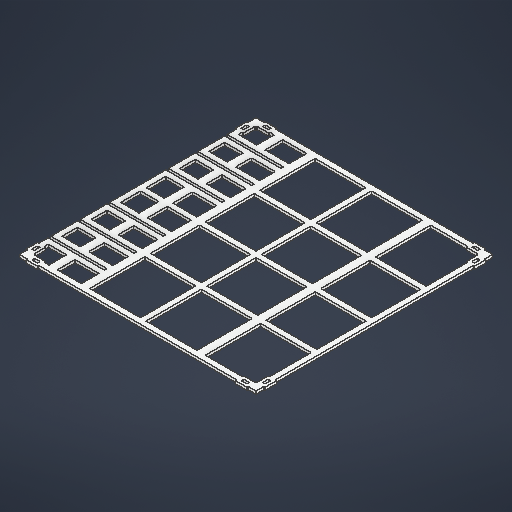
# Autodesk Inventor part: seat
Saved by Autodesk Inventor 2027.1 (Build 311270010, 270A)
## iProperties
Created: 2025-09-19
Part Number: seat
Material: Foam Core Board
Document SubType Name: Modeling
Designer: Nick
Density: 0.141998 g/cm^3
Appearance: Default(1)
Mass: 39.809 g
Surface Area: 1606.94 cm^2
Volume: 280.349 cm^3
Author: Nick
Autodesk Inventor part; units mm, degrees
ref_plane "YZ Plane" through (0, 0, 0) normal (1, 0, 0) x (0, 1, 0)
ref_plane "XZ Plane" through (0, 0, 0) normal (0, 1, 0) x (-1, 0, 0)
ref_plane "XY Plane" through (0, 0, 0) normal (0, 0, 1) x (1, 0, 0)
sketch "Sketch11" plane through (0, 0, 0) normal (0, 1, 0) x (-1, 0, 0)
  line L0 (0, 0) -> (420.5, 0)
  line L1 (420.5, 0) -> (420.5, -420.5)
  line L2 (420.5, -420.5) -> (0, -420.5)
  line L3 (0, -420.5) -> (0, 0)
  line L4 (420.5, 0) -> (410.5, 0)
  line L5 (410.5, 0) -> (410.5, -10)
  line L6 (410.5, -10) -> (420.5, -10)
  line L7 (420.5, -10) -> (420.5, 0)
  line L8 (0, -420.5) -> (10, -420.5)
  line L9 (10, -420.5) -> (10, -410.5)
  line L10 (10, -410.5) -> (0, -410.5)
  line L11 (0, -410.5) -> (0, -420.5)
  line L12 (10, -410.5) -> (410.5, -410.5)
  line L13 (410.5, -410.5) -> (410.5, -10)
  line L14 (410.5, -10) -> (10, -10)
  line L15 (10, -10) -> (10, -410.5)
  line L16 (0, -46.5229) -> (115, -46.5229)
  line L17 (115, -10) -> (100, -10)
  line L18 (100, -10) -> (100, -410.5)
  line L19 (100, -410.5) -> (115, -410.5)
  line L20 (115, -410.5) -> (115, -10)
  line L21 (210.25, 0) -> (210.25, -567.6903)
  line L22 (305.5, -10) -> (320.5, -10)
  line L23 (320.5, -10) -> (320.5, -410.5)
  line L24 (320.5, -410.5) -> (305.5, -410.5)
  line L25 (305.5, -410.5) -> (305.5, -10)
  line L26 (420.5, -210.25) -> (420.5, -205.25)
  line L27 (420.5, -205.25) -> (0, -205.25)
  line L28 (0, -205.25) -> (0, -215.25)
  line L29 (0, -215.25) -> (420.5, -215.25)
  line L30 (420.5, -215.25) -> (420.5, -205.25)
  line L31 (210.25, -420.5) -> (215.25, -420.5)
  line L32 (215.25, -420.5) -> (205.25, -420.5)
  line L33 (205.25, -420.5) -> (205.25, -10)
  line L34 (205.25, -10) -> (215.25, -10)
  line L35 (215.25, -10) -> (215.25, -420.5)
  point P0 (305.5, -46.5229)
  point P1 (410.5, -205.25)
  point P2 (320.5, -205.25)
  point P3 (10, -205.25)
  point P4 (205.25, -205.25)
  point P5 (410.5, -215.25)
  point P6 (320.5, -215.25)
  point P7 (305.5, -205.25)
  point P8 (215.25, -205.25)
  point P9 (305.5, -215.25)
  point P10 (215.25, -410.5)
  point P11 (215.25, -215.25)
  point P12 (10, -215.25)
  point P13 (205.25, -215.25)
  point P14 (205.25, -410.5)
  point P15 (100, -205.25)
  point P16 (115, -205.25)
  point P17 (115, -215.25)
  point P18 (100, -215.25)
  dimension "d88" = 420.5
  dimension "d89" = 420.5
  dimension "d90" = 10
  dimension "d91" = 10
  dimension "d92" = 10
  dimension "d93" = 10
  dimension "d94" = 115
  dimension "d95" = 15
  dimension "d96" = 5
  dimension "d97" = 10
  dimension "d98" = 5
  dimension "d99" = 10
  constraints: 72 end point, 14 parallel, 8 horizontal, 8 point on line, 7 perpendicular, 5 symmetric about line, 3 midpoint, 1 vertical
  measures "d88" distance of L1.end L2.end
  measures "d89" distance of L0.end L1.end
  measures "d90" distance of L6.end L5.end
  measures "d91" distance of L5.end L4.end
  measures "d92" distance of L10.end L9.end
  measures "d93" distance of L9.end L8.end
  measures "d94" distance of L16.start L16.end
  measures "d95" distance of L19.end L18.end
  measures "d96" distance of L26.start L26.end
  measures "d97" distance of L28.end L27.end
  measures "d98" distance of L31.start L31.end
  measures "d99" distance of L33.end L34.end
extrude "Extrusion12" add sketch "Sketch11" along normal blind 5 contours L0 L21 L14 L15 L16 L3 | L0 L5 L14 L21 | L16 L15 L27 L3 | L0 L1 L6 L5 | L21 L27 L33 L14 | L14 L35 L27 L21 | L27 L15 L29 L3 | L6 L1 L27 L13 | L27 L35 L29 L21 | L21 L29 L33 L27 | L29 L15 L10 L3 | L27 L18 L29 L15 | L18 L14 L20 L16 | L16 L20 L27 L18 | L27 L1 L29 L13 | L13 L29 L23 L27 | L23 L27 L25 L14 | L27 L25 L29 L35 | L33 L29 L20 L27 | L29 L35 L12 L21 | L21 L12 L33 L29 | L10 L9 L2 L3 | L27 L20 L29 L18 | L29 L1 L2 L35 L12 L13 | L23 L29 L25 L27 | L21 L2 L33 L12 | L12 L35 L2 L21 | L12 L33 L2 L9 | L29 L20 L12 L18 | L23 L12 L25 L29
sketch "Sketch12" plane through (0, 5, 0) normal (0, 1, 0) x (1, 0, 0)
  line L0 (-420.5, 420.5) -> (-420.5, 0) projected
  line L1 (-420.5, 0) -> (-420.5, 51.25)
  line L2 (-420.5, 51.25) -> (-320.5, 51.25)
  line L3 (-320.5, 51.25) -> (-320.5, 55.75)
  line L4 (-320.5, 55.75) -> (-420.5, 55.75)
  line L5 (-420.5, 51.25) -> (-420.5, 41.25)
  line L6 (-420.5, 41.25) -> (-320.5, 41.25)
  line L7 (-320.5, 41.25) -> (-320.5, 51.25)
  line L8 (-320.5, 205.25) -> (-320.5, 10) projected
  line L9 (-320.5, 55.75) -> (-320.5, 65.75)
  line L10 (-320.5, 65.75) -> (-420.5, 65.75)
  line L11 (-420.5, 65.75) -> (-420.5, 55.75)
  line L12 (-420.5, 55.75) -> (-420.5, 51.25)
  line L13 (-320.5, 51.25) -> (-320.5, 55.75)
  line L14 (-370.5, 10) -> (-378, 10)
  line L15 (-320.5, 10) -> (-410.5, 10) projected
  line L16 (-410.5, 410.5) -> (-320.5, 410.5) projected
  line L17 (-378, 10) -> (-363, 10)
  line L18 (-363, 10) -> (-363, 410.5)
  line L19 (-363, 410.5) -> (-378, 410.5)
  line L20 (-378, 410.5) -> (-378, 10)
  line L21 (-320.5, 103.5) -> (-320.5, 108)
  line L22 (-320.5, 103.5) -> (-320.5, 108)
  line L23 (-320.5, 93.5) -> (-320.5, 103.5)
  line L24 (-320.5, 108) -> (-320.5, 118)
  line L25 (-420.5, 103.5) -> (-320.5, 103.5)
  line L26 (-420.5, 108) -> (-420.5, 103.5)
  line L27 (-320.5, 108) -> (-420.5, 108)
  line L28 (-420.5, 103.5) -> (-420.5, 93.5)
  line L29 (-420.5, 93.5) -> (-320.5, 93.5)
  line L30 (-420.5, 118) -> (-420.5, 108)
  line L31 (-320.5, 118) -> (-420.5, 118)
  line L32 (-320.5, 155.75) -> (-320.5, 160.25)
  line L33 (-320.5, 155.75) -> (-320.5, 160.25)
  line L34 (-320.5, 145.75) -> (-320.5, 155.75)
  line L35 (-320.5, 160.25) -> (-320.5, 170.25)
  line L36 (-420.5, 155.75) -> (-320.5, 155.75)
  line L37 (-420.5, 160.25) -> (-420.5, 155.75)
  line L38 (-320.5, 160.25) -> (-420.5, 160.25)
  line L39 (-420.5, 155.75) -> (-420.5, 145.75)
  line L40 (-420.5, 145.75) -> (-320.5, 145.75)
  line L41 (-420.5, 170.25) -> (-420.5, 160.25)
  line L42 (-320.5, 170.25) -> (-420.5, 170.25)
  line L43 (-420.5, 210.25) -> (40.6434, 210.25)
  line L44 (-420.5, 420.5) -> (-420.5, 369.25)
  line L45 (-420.5, 369.25) -> (-320.5, 369.25)
  line L46 (-320.5, 369.25) -> (-320.5, 364.75)
  line L47 (-320.5, 364.75) -> (-420.5, 364.75)
  line L48 (-420.5, 369.25) -> (-420.5, 379.25)
  line L49 (-420.5, 379.25) -> (-320.5, 379.25)
  line L50 (-320.5, 379.25) -> (-320.5, 369.25)
  line L51 (-320.5, 364.75) -> (-320.5, 354.75)
  line L52 (-320.5, 354.75) -> (-420.5, 354.75)
  line L53 (-420.5, 354.75) -> (-420.5, 364.75)
  line L54 (-420.5, 364.75) -> (-420.5, 369.25)
  line L55 (-320.5, 369.25) -> (-320.5, 364.75)
  line L56 (-370.5, 410.5) -> (-378, 410.5)
  line L57 (-320.5, 410.5) -> (-410.5, 410.5)
  line L58 (-378, 410.5) -> (-363, 410.5)
  line L59 (-320.5, 317) -> (-320.5, 312.5)
  line L60 (-320.5, 317) -> (-320.5, 312.5)
  line L61 (-320.5, 327) -> (-320.5, 317)
  line L62 (-320.5, 312.5) -> (-320.5, 302.5)
  line L63 (-420.5, 317) -> (-320.5, 317)
  line L64 (-420.5, 312.5) -> (-420.5, 317)
  line L65 (-320.5, 312.5) -> (-420.5, 312.5)
  line L66 (-420.5, 317) -> (-420.5, 327)
  line L67 (-420.5, 327) -> (-320.5, 327)
  line L68 (-420.5, 302.5) -> (-420.5, 312.5)
  line L69 (-320.5, 302.5) -> (-420.5, 302.5)
  line L70 (-320.5, 264.75) -> (-320.5, 260.25)
  line L71 (-320.5, 264.75) -> (-320.5, 260.25)
  line L72 (-320.5, 274.75) -> (-320.5, 264.75)
  line L73 (-320.5, 260.25) -> (-320.5, 250.25)
  line L74 (-420.5, 264.75) -> (-320.5, 264.75)
  line L75 (-420.5, 260.25) -> (-420.5, 264.75)
  line L76 (-320.5, 260.25) -> (-420.5, 260.25)
  line L77 (-420.5, 264.75) -> (-420.5, 274.75)
  line L78 (-420.5, 274.75) -> (-320.5, 274.75)
  line L79 (-420.5, 250.25) -> (-420.5, 260.25)
  line L80 (-320.5, 250.25) -> (-420.5, 250.25)
  line L81 (-420.5, 274.75) -> (-420.5, 250.25)
  line L82 (-420.5, 274.75) -> (-378, 274.75)
  line L83 (-378, 264.75) -> (-420.5, 264.75)
  line L84 (-378, 260.25) -> (-420.5, 260.25)
  line L85 (-378, 312.5) -> (-420.5, 312.5)
  line L86 (-420.5, 317) -> (-378, 317)
  line L87 (-410.5, 215.25) -> (-410.5, 410.5) projected
  line L88 (-410.5, 302.5) -> (-410.5, 274.75)
  point P0 (0, 0)
  point P1 (-363, 93.5)
  point P2 (-363, 103.5)
  point P3 (-363, 108)
  point P4 (-363, 118)
  point P5 (-363, 145.75)
  point P6 (-363, 155.75)
  point P7 (-363, 160.25)
  point P8 (-363, 170.25)
  point P9 (-378, 170.25)
  point P10 (-378, 145.75)
  point P11 (-378, 118)
  point P12 (-378, 108)
  point P13 (-378, 103.5)
  point P14 (-378, 93.5)
  point P15 (-378, 55.75)
  point P16 (-378, 51.25)
  point P17 (-363, 51.25)
  point P18 (-363, 55.75)
  point P19 (-378, 354.75)
  point P20 (-378, 364.75)
  point P21 (-378, 379.25)
  point P22 (-378, 369.25)
  point P23 (-363, 379.25)
  point P24 (-363, 369.25)
  point P25 (-363, 364.75)
  point P26 (-363, 354.75)
  point P27 (-363, 312.5)
  point P28 (-363, 302.5)
  point P29 (-363, 327)
  point P30 (-363, 317)
  point P31 (-363, 260.25)
  point P32 (-363, 250.25)
  point P33 (-363, 274.75)
  point P34 (-363, 264.75)
  point P35 (-378, 250.25)
  point P36 (-378, 327)
  point P37 (-378, 302.5)
  dimension "d102" = 51.25
  dimension "d103" = 100
  dimension "d104" = 4.5
  dimension "d105" = 10
  dimension "d106" = 10
  dimension "d111" = 7.5
  dimension "d112" = 15
  dimension "d115" = 52.25
  constraints: 164 end point, 27 point on line, 25 symmetric about line, 21 collinear, 16 vertical alignment, 9 parallel, 5 perpendicular, 3 horizontal, 15 other
  measures "d102" distance of L1.start L1.end
  measures "d103" distance of L1.end L2.end
  measures "d104" distance of L2.end L3.end
  measures "d105" distance of L1.end L5.end
  measures "d106" distance of L3.end L9.end
  measures "d111" distance of L14.start L14.end
  measures "d112" distance of L19.end L19.start
  measures "d115" distance of L3.end L21.end
extrude "Extrusion13" add sketch "Sketch12" against normal blind 5 contours L10 L20 L4 L0 | L10 L18 L4 L20 | L2 L20 L6 L0 | L10 L8 L4 L18 | L2 L18 L6 L20 | L2 L7 L6 L18
extrude "Extrusion14" cut sketch "Sketch12" against normal blind 5 contours L38 L20 L36 L0 | L38 L18 L36 L20 | L38 L8 L36 L18 | L27 L20 L25 L0 | L27 L18 L25 L20 | L27 L8 L25 L18 | L4 L20 L2 L0 | L4 L18 L2 L20 | L4 L3 L2 L18
extrude "Extrusion15" add sketch "Sketch12" against normal blind 5 contours L49 L87 L45 L0 | L49 L20 L45 L87 | L47 L87 L52 L0 | L49 L18 L45 L20 | L20 L16 L18 L49 | L47 L20 L52 L87 | L45 L18 L47 L20 | L49 L50 L45 L18 | L67 L87 L63 L0 | L47 L18 L52 L20 | L63 L87 L65 L0 | L67 L20 L63 L87 | L52 L18 L67 L20 | L47 L51 L52 L18 | L65 L87 L69 L0 | L63 L20 L65 L87 | L67 L18 L63 L20 | L69 L87 L78 L0 | L65 L20 L69 L87 | L63 L18 L65 L20 | L67 L61 L63 L18 | L78 L87 L74 L0 | L69 L20 L78 L87 | L65 L18 L69 L20 | L74 L87 L76 L0 | L78 L20 L74 L87 | L69 L18 L78 L20 | L65 L62 L69 L18 | L76 L87 L80 L0 | L74 L20 L76 L87 | L78 L18 L74 L20 | L76 L20 L80 L87 | L74 L18 L76 L20 | L78 L72 L74 L18 | L76 L18 L80 L20 | L42 L20 L38 L0 | L43 L18 L42 L20 | L20 L80 L18 L43 | L76 L73 L80 L18 | L38 L20 L36 L0 | L42 L18 L38 L20 | L36 L20 L40 L0 | L38 L18 L36 L20 | L42 L8 L38 L18 | L36 L18 L40 L20 | L31 L20 L27 L0 | L40 L18 L31 L20 | L36 L8 L40 L18 | L31 L18 L27 L20 | L25 L20 L29 L0 | L27 L18 L25 L20 | L31 L8 L27 L18 | L25 L18 L29 L20 | L29 L18 L10 L20 | L25 L8 L29 L18 | L10 L18 L4 L20 | L4 L18 L2 L20 | L2 L18 L6 L20 | L6 L18 L15 L14 L20
extrude "Extrusion16" cut sketch "Sketch12" against normal blind 5 contours L38 L20 L36 L0 | L38 L18 L36 L20 | L27 L18 L25 L20 | L4 L18 L2 L20
extrude "Extrusion17" cut sketch "Sketch12" against normal blind 5 contours L45 L87 L47 L0 | L45 L20 L47 L87 | L45 L18 L47 L20 | L63 L87 L65 L0 | L63 L20 L65 L87 | L63 L18 L65 L20 | L69 L20 L78 L87 | L74 L87 L76 L0 | L74 L20 L76 L87 | L74 L18 L76 L20
sketch "Sketch13" plane through (0, 5, 0) normal (0, 1, 0) x (1, 0, 0)
  line L0 (0, 0) -> (0, 420.5) projected
  line L1 (-320.5, 108) -> (0, 108)
  line L2 (0, 108) -> (0, 118)
  line L3 (0, 118) -> (-320.5, 118)
  line L4 (-320.5, 118) -> (-320.5, 108)
  line L5 (-420.5, 260.25) -> (-420.5, 160.25) projected
  line L6 (-420.5, 210.25) -> (46.3484, 210.25)
  line L7 (-320.5, 312.5) -> (0, 312.5)
  line L8 (0, 312.5) -> (0, 302.5)
  line L9 (0, 302.5) -> (-320.5, 302.5)
  line L10 (-320.5, 302.5) -> (-320.5, 312.5)
  dimension "d126" = 10
  constraints: 18 end point, 4 symmetric about line, 2 horizontal, 2 parallel, 1 midpoint, 1 perpendicular, 1 point on line
  measures "d126" distance of L2.end L1.end
extrude "Extrusion18" add sketch "Sketch13" against normal blind 5
sketch "Sketch14" plane through (0, 5, 0) normal (0, 1, 0) x (1, 0, 0)
  line L0 (-420.5, 0) -> (0, 0) projected
  line L1 (0, 0) -> (-19.25, 0)
  line L2 (-19.25, 0) -> (-19.25, 2.75)
  line L3 (-19.25, 2.75) -> (-29.25, 2.75)
  line L4 (-29.25, 2.75) -> (-29.25, 7.25)
  line L5 (-29.25, 7.25) -> (-19.25, 7.25)
  line L6 (-19.25, 7.25) -> (-19.25, 2.75)
  line L7 (0, 0) -> (0, 19.25)
  line L8 (0, 0) -> (0, 420.5) projected
  line L9 (0, 19.25) -> (-2.75, 19.25)
  line L10 (-2.75, 19.25) -> (-7.25, 19.25)
  line L11 (-7.25, 19.25) -> (-7.25, 29.25)
  line L12 (-7.25, 29.25) -> (-2.75, 29.25)
  line L13 (-2.75, 29.25) -> (-2.75, 19.25)
  line L14 (-29.25, 2.75) -> (-29.25, -2.25)
  line L15 (-29.25, -2.25) -> (-34.25, -2.25)
  line L16 (-19.25, 7.25) -> (-19.25, 12.25)
  line L17 (-19.25, 12.25) -> (-14.25, 12.25)
  line L18 (-7.25, 19.25) -> (-12.25, 19.25)
  line L19 (-12.25, 19.25) -> (-12.25, 14.25)
  line L20 (-2.75, 29.25) -> (-2.75, 34.25)
  line L21 (-2.75, 34.25) -> (2.25, 34.25)
  line L22 (-34.25, -2.25) -> (-14.25, -2.25)
  line L23 (-14.25, -2.25) -> (-14.25, 12.25)
  line L24 (-14.25, 12.25) -> (-34.25, 12.25)
  line L25 (-34.25, 12.25) -> (-34.25, -2.25)
  line L26 (-12.25, 14.25) -> (2.25, 14.25)
  line L27 (2.25, 14.25) -> (2.25, 34.25)
  line L28 (2.25, 34.25) -> (-12.25, 34.25)
  line L29 (-12.25, 34.25) -> (-12.25, 14.25)
  line L30 (-10, 10) -> (-100, 10) projected
  line L31 (-10, 10) -> (-14.25, 10)
  line L32 (-14.25, 10) -> (-14.25, 14.25)
  line L33 (-14.25, 14.25) -> (-10, 14.25)
  line L34 (-10, 14.25) -> (-10, 10)
  line L35 (0, 210.25) -> (-440.8784, 210.25)
  line L36 (-210.25, 0) -> (-210.25, 464.0393)
  line L37 (0, 420.5) -> (-19.25, 420.5)
  line L38 (-19.25, 420.5) -> (-19.25, 417.75)
  line L39 (-19.25, 417.75) -> (-29.25, 417.75)
  line L40 (-29.25, 417.75) -> (-29.25, 413.25)
  line L41 (-29.25, 413.25) -> (-19.25, 413.25)
  line L42 (-19.25, 413.25) -> (-19.25, 417.75)
  line L43 (0, 420.5) -> (0, 401.25)
  line L44 (0, 401.25) -> (-2.75, 401.25)
  line L45 (-2.75, 401.25) -> (-7.25, 401.25)
  line L46 (-7.25, 401.25) -> (-7.25, 391.25)
  line L47 (-7.25, 391.25) -> (-2.75, 391.25)
  line L48 (-2.75, 391.25) -> (-2.75, 401.25)
  line L49 (-29.25, 417.75) -> (-29.25, 422.75)
  line L50 (-29.25, 422.75) -> (-34.25, 422.75)
  line L51 (-19.25, 413.25) -> (-19.25, 408.25)
  line L52 (-19.25, 408.25) -> (-14.25, 408.25)
  line L53 (-7.25, 401.25) -> (-12.25, 401.25)
  line L54 (-12.25, 401.25) -> (-12.25, 406.25)
  line L55 (-2.75, 391.25) -> (-2.75, 386.25)
  line L56 (-2.75, 386.25) -> (2.25, 386.25)
  line L57 (-34.25, 422.75) -> (-14.25, 422.75)
  line L58 (-14.25, 422.75) -> (-14.25, 408.25)
  line L59 (-14.25, 408.25) -> (-34.25, 408.25)
  line L60 (-34.25, 408.25) -> (-34.25, 422.75)
  line L61 (-12.25, 406.25) -> (2.25, 406.25)
  line L62 (2.25, 406.25) -> (2.25, 386.25)
  line L63 (2.25, 386.25) -> (-12.25, 386.25)
  line L64 (-12.25, 386.25) -> (-12.25, 406.25)
  line L65 (-10, 410.5) -> (-14.25, 410.5)
  line L66 (-14.25, 410.5) -> (-14.25, 406.25)
  line L67 (-14.25, 406.25) -> (-10, 406.25)
  line L68 (-10, 406.25) -> (-10, 410.5)
  line L69 (-420.5, 0) -> (-401.25, 0)
  line L70 (-401.25, 0) -> (-401.25, 2.75)
  line L71 (-401.25, 2.75) -> (-391.25, 2.75)
  line L72 (-391.25, 2.75) -> (-391.25, 7.25)
  line L73 (-391.25, 7.25) -> (-401.25, 7.25)
  line L74 (-401.25, 7.25) -> (-401.25, 2.75)
  line L75 (-420.5, 0) -> (-420.5, 19.25)
  line L76 (-420.5, 0) -> (-420.5, 420.5)
  line L77 (-420.5, 19.25) -> (-417.75, 19.25)
  line L78 (-417.75, 19.25) -> (-413.25, 19.25)
  line L79 (-413.25, 19.25) -> (-413.25, 29.25)
  line L80 (-413.25, 29.25) -> (-417.75, 29.25)
  line L81 (-417.75, 29.25) -> (-417.75, 19.25)
  line L82 (-391.25, 2.75) -> (-391.25, -2.25)
  line L83 (-391.25, -2.25) -> (-386.25, -2.25)
  line L84 (-401.25, 7.25) -> (-401.25, 12.25)
  line L85 (-401.25, 12.25) -> (-406.25, 12.25)
  line L86 (-413.25, 19.25) -> (-408.25, 19.25)
  line L87 (-408.25, 19.25) -> (-408.25, 14.25)
  line L88 (-417.75, 29.25) -> (-417.75, 34.25)
  line L89 (-417.75, 34.25) -> (-422.75, 34.25)
  line L90 (-386.25, -2.25) -> (-406.25, -2.25)
  line L91 (-406.25, -2.25) -> (-406.25, 12.25)
  line L92 (-406.25, 12.25) -> (-386.25, 12.25)
  line L93 (-386.25, 12.25) -> (-386.25, -2.25)
  line L94 (-408.25, 14.25) -> (-422.75, 14.25)
  line L95 (-422.75, 14.25) -> (-422.75, 34.25)
  line L96 (-422.75, 34.25) -> (-408.25, 34.25)
  line L97 (-408.25, 34.25) -> (-408.25, 14.25)
  line L98 (-410.5, 10) -> (-406.25, 10)
  line L99 (-406.25, 10) -> (-406.25, 14.25)
  line L100 (-406.25, 14.25) -> (-410.5, 14.25)
  line L101 (-410.5, 14.25) -> (-410.5, 10)
  line L102 (-420.5, 420.5) -> (-401.25, 420.5)
  line L103 (-401.25, 420.5) -> (-401.25, 417.75)
  line L104 (-401.25, 417.75) -> (-391.25, 417.75)
  line L105 (-413.25, 391.25) -> (-417.75, 391.25)
  line L106 (-417.75, 391.25) -> (-417.75, 386.25)
  line L107 (-420.5, 401.25) -> (-417.75, 401.25)
  line L108 (-413.25, 401.25) -> (-408.25, 401.25)
  line L109 (-417.75, 391.25) -> (-417.75, 401.25)
  line L110 (-408.25, 386.25) -> (-408.25, 406.25)
  line L111 (-401.25, 408.25) -> (-406.25, 408.25)
  line L112 (-406.25, 410.5) -> (-406.25, 406.25)
  line L113 (-391.25, 413.25) -> (-401.25, 413.25)
  line L114 (-401.25, 413.25) -> (-401.25, 408.25)
  line L115 (-391.25, 417.75) -> (-391.25, 413.25)
  line L116 (-401.25, 413.25) -> (-401.25, 417.75)
  line L117 (-420.5, 420.5) -> (-420.5, 401.25)
  line L118 (-413.25, 401.25) -> (-413.25, 391.25)
  line L119 (-417.75, 401.25) -> (-413.25, 401.25)
  line L120 (-391.25, 417.75) -> (-391.25, 422.75)
  line L121 (-391.25, 422.75) -> (-386.25, 422.75)
  line L122 (-408.25, 401.25) -> (-408.25, 406.25)
  line L123 (-406.25, 408.25) -> (-386.25, 408.25)
  line L124 (-410.5, 410.5) -> (-406.25, 410.5)
  line L125 (-406.25, 406.25) -> (-410.5, 406.25)
  line L126 (-410.5, 406.25) -> (-410.5, 410.5)
  line L127 (-417.75, 386.25) -> (-422.75, 386.25)
  line L128 (-422.75, 406.25) -> (-422.75, 386.25)
  line L129 (-422.75, 386.25) -> (-408.25, 386.25)
  line L130 (-408.25, 406.25) -> (-422.75, 406.25)
  line L131 (-386.25, 422.75) -> (-406.25, 422.75)
  line L132 (-386.25, 408.25) -> (-386.25, 422.75)
  line L133 (-406.25, 422.75) -> (-406.25, 408.25)
  point P0 (-420.5, 210.25)
  dimension "d129" = 19.25
  dimension "d130" = 2.75
  dimension "d131" = 10
  dimension "d132" = 4.5
  dimension "d135" = 19.25
  dimension "d136" = 2.75
  dimension "d137" = 4.5
  dimension "d138" = 10
  dimension "d139" = 5
  dimension "d140" = 5
  dimension "d141" = 5
  dimension "d142" = 5
  dimension "d143" = 5
  dimension "d144" = 5
  dimension "d145" = 5
  dimension "d146" = 5
  constraints: 262 end point, 80 symmetric about line, 11 perpendicular, 11 point on line, 10 parallel, 7 horizontal, 4 vertical, 2 midpoint
  measures "d129" distance of L0.end L1.end
  measures "d130" distance of L1.end L2.end
  measures "d131" distance of L4.end L5.end
  measures "d132" distance of L3.end L4.end
  measures "d135" distance of L0.end L7.end
  measures "d136" distance of L7.end L9.end
  measures "d137" distance of L11.end L12.end
  measures "d138" distance of L10.end L11.end
  measures "d139" distance of L3.end L14.end
  measures "d140" distance of L14.end L15.end
  measures "d141" distance of L5.end L16.end
  measures "d142" distance of L16.end L17.end
  measures "d143" distance of L10.end L18.end
  measures "d144" distance of L18.end L19.end
  measures "d145" distance of L12.end L20.end
  measures "d146" distance of L20.end L21.end
extrude "Extrusion19" cut sketch "Sketch14" against normal blind 5 contours L74 L73 L72 L71 | L81 L80 L79 L78 | L119 L118 L105 L109 | L4 L5 L6 L3 | L10 L11 L12 L13 | L48 L47 L46 L45 | L104 L115 L113 L116 | L42 L41 L40 L39
extrude "Extrusion20" add sketch "Sketch14" against normal blind 5 contours L127 L128 L130 L76 | L76 L107 L109 L106 L127 | L56 L55 L48 L44 L8 | L8 L61 L62 L56 | L91 L85 L84 L74 L70 L0 | L0 L82 L90 L91 | L94 L95 L89 L76 L75 | L75 L77 L78 L86 L87 L94 | L70 L71 L82 L0 | L98 L101 L94 L100 L99 L91 | L76 L89 L88 L81 L77 | L82 L72 L73 L84 L92 L93 L0 | L0 L93 L83 L82 | L96 L97 L86 L79 L80 L88 | L25 L30 L16 L5 L4 L14 L0 | L0 L14 L15 L25 | L76 L130 L125 L110 L108 L119 L107 | L106 L105 L118 L108 L110 L129 | L14 L3 L2 L0 | L0 L23 L22 L14 | L25 L24 L16 L30 | L21 L27 L26 L7 L8 | L8 L9 L13 L20 L21 | L2 L6 L16 L30 L23 L0 | L16 L17 L23 L30 | L7 L26 L19 L18 L10 L9 | L20 L12 L11 L18 L29 L28 | L44 L45 L53 L54 L61 L8 | L63 L64 L53 L46 L47 L55 | L126 L124 L112 L125 | L23 L32 L33 L26 L34 L30 | L133 L131 L120 L104 L103 L102 | L102 L103 L116 L114 L111 L112 L133 | L61 L67 L66 L58 L65 L68 | L58 L52 L51 L42 L38 L37 | L37 L38 L39 L49 L57 L58 | L121 L132 L123 L114 L113 L115 L120 | L49 L40 L41 L51 L59 L60 L50
body "Solid2"
